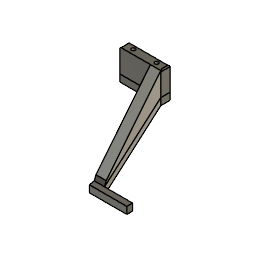
Aeolus Task 2 (Autodesk Fusion 360 design; units mm, degrees)
part number: 2026-09-11-21-48-32-788
part number: 2026-09-11-21-49-10-979
Autodesk Fusion 360 part; units mm, degrees
sketch "Sketch1" plane through (0, 0, 0) normal (0, 0, 1) x (1, 0, 0)
  line L0 (0, 0) -> (35, 0)
  line L1 (35, 0) -> (35, -8)
  line L2 (35, -8) -> (76.9677, -98)
  line L3 (76.9677, -98) -> (100.9677, -98)
  line L4 (100.9677, -98) -> (100.9677, -103)
  line L5 (100.9677, -103) -> (68.9677, -103)
  line L6 (68.9677, -103) -> (68.1407, -98)
  line L7 (68.1407, -98) -> (26.173, -8)
  line L8 (26.173, -8) -> (0, -8)
  line L9 (0, -8) -> (0, 0)
  circle A0 centre (7.5, -4) radius 1.6
  circle A1 centre (27.5, -4) radius 1.6
extrude "Extrude1" add sketch "Sketch1" along normal mid plane 6 makes body 1
extrude "Extrude1'" add 1 faces at (43.1045, -38, 3) along direction (0, 0, 1) blind 20 separate body on bodies 1 makes body 2 in component "Component"
sketch "Sketch2" plane through (0, 0, 23) normal (0, 0, 1) x (-1, 0, 0)
  circle A0 centre (-7.5, 4) radius 1.6
  circle A1 centre (-27.5, 4) radius 1.6
  line L0 (0, 8) -> (-26.173, 8)
  line L1 (-26.173, 8) -> (-68.1407, 98)
  line L2 (-68.1407, 98) -> (-68.9677, 103)
  line L3 (-68.9677, 103) -> (-100.9677, 103)
  line L4 (-100.9677, 103) -> (-100.9677, 98)
  line L5 (-100.9677, 98) -> (-76.9677, 98)
  line L6 (-76.9677, 98) -> (-35, 8)
  line L7 (-35, 8) -> (-35, 0)
  line L8 (-35, 0) -> (0, 0)
  line L9 (0, 0) -> (0, 8)
  line L10 (-100.9677, 98) -> (-68.9677, 98)
  line L11 (-68.9677, 98) -> (-68.9677, 103)
  line L12 (-68.9677, 103) -> (-100.9677, 103)
  line L13 (-100.9677, 103) -> (-100.9677, 98)
  constraint horizontal L10
  constraint vertical L11
  constraint horizontal L12
  constraint vertical L13
  constraint coincident L2.end L3.start
  constraint coincident L4.end L5.start
extrude "Extrude2" cut sketch "Sketch2" against normal blind 20 contours L3 L4 L5 L10 L11 L12 L13 bodies 2 in component "Component"
sketch "Sketch3" plane through (0, 0, 23) normal (0, 0, 1) x (-1, 0, 0)
  line L0 (-68.9677, 98) -> (-76.9677, 98)
  line L1 (-76.9677, 98) -> (-35, 8)
  line L2 (-35, 8) -> (-35, 0)
  line L3 (-35, 0) -> (0, 0)
  line L4 (0, 0) -> (0, 8)
  line L5 (0, 8) -> (-26.173, 8)
  line L6 (-26.173, 8) -> (-68.1407, 98)
  line L7 (-68.1407, 98) -> (-68.9677, 103)
  line L8 (-68.9677, 103) -> (-68.9677, 98)
  circle A0 centre (-7.5, 4) radius 1.6
  circle A1 centre (-27.5, 4) radius 1.6
  line L9 (-68.9677, 98) -> (-68.1407, 98)
  line L10 (-68.9677, 103) -> (-68.9677, 98)
  constraint coincident L0.start L8.end
  constraint coincident L6.end L7.start
  constraint coincident L7.end L8.start
extrude "Extrude3" cut sketch "Sketch3" against normal blind 20 contours L7 L8 L9 L10 bodies 2 in component "Component"
chamfer "Chamfer1" distance 20 angle 45 1 edges at (72.5542, -98, 23) on bodies 2 in component "Component"
chamfer "Chamfer2" distance 25 angle 45 1 edges at (63.228, -78, 23) on bodies 2 in component "Component"
chamfer "Chamfer3" distance 45 angle 45 1 edges at (51.5703, -53, 23) on bodies 2 in component "Component"
delete_face "DeleteFace1" 1 faces at (72.771, -95.31, 5.4746) on bodies 2 in component "Component"
fillet "Fillet1" radius 1 3 edges at (35, -4, 23) (17.5, 0, 23) (0, -4, 23) on bodies 2 in component "Component"
component "Component" placed x (1, 0, 0) y (0, 1, 0) z (0, 0, 1) at (0, 0, 0)
